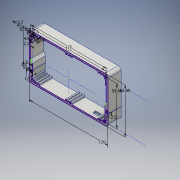
# Autodesk Inventor part: SZOMK-AK-C-C39
Saved by Autodesk Inventor 2016 (Build 200138000, 138)
## iProperties
Created: 2016-04-01
Part Number: SZOMK-AK-C-C39
Material: Aluminum 6061
Document SubType Name: Modeling
Designer: admin
Density: 2.7 g/cm^3
Appearance: Aluminum - Flat
Author: admin
Autodesk Inventor part; units mm, degrees
ref_plane "YZ Plane" through (0, 0, 0) normal (1, 0, 0) x (0, 1, 0)
ref_plane "XZ Plane" through (0, 0, 0) normal (0, 1, 0) x (-1, 0, 0)
ref_plane "XY Plane" through (0, 0, 0) normal (0, 0, 1) x (1, 0, 0)
sketch "Sketch1" plane through (0, 0, 0) normal (0, 1, 0) x (-1, 0, 0)
  arc A0 (55.1118, 28.4761) -> (54.0511, 29.5368) centre (55.5, 29.925) ccw
  arc A1 (-54.0059, 29.7916) -> (-55.1118, 28.4761) centre (-55.5, 29.925) ccw
  arc A2 (54.0511, -29.5368) -> (55.1118, -28.4761) centre (55.5, -29.925) ccw
  arc A3 (-55.1118, -28.4761) -> (-54.0511, -29.5368) centre (-55.5, -29.925) ccw
  line L0 (55.5, 34.425) -> (-55.5, 34.425)
  line L1 (55.5, -34.425) -> (-55.5, -34.425)
  line L2 (33.1179, 0) -> (-42.957, 0) construction
  line L3 (0, -20.0068) -> (0, 12.0803) construction
  line L4 (-77.7331, -29.925) -> (-117.8042, -29.925) construction
  line L5 (-91.6184, 29.925) -> (-122.9166, 29.925) construction
  line L6 (55.5, -18.8016) -> (55.5, 12.0803) construction
  line L7 (-55.5, -18.8016) -> (-55.5, 16.5996) construction
  arc A4 (55.5, -34.425) -> (60, -29.925) centre (55.5, -29.925) ccw
  arc A5 (60, 29.925) -> (55.5, 34.425) centre (55.5, 29.925) ccw
  arc A6 (-55.5, 34.425) -> (-60, 29.925) centre (-55.5, 29.925) ccw
  arc A7 (-60, -29.925) -> (-55.5, -34.425) centre (-55.5, -29.925) ccw
  line L8 (57.5, 27.125) -> (57.5, 25.125)
  line L9 (57.5, 25.125) -> (55.5, 25.125)
  line L10 (55.5, 25.125) -> (55.5, 23.125)
  line L11 (55.5, 23.125) -> (57.5, 23.125)
  line L12 (57.5, 23.125) -> (57.5, 21.125)
  line L13 (57.5, 21.125) -> (55.5, 21.125)
  line L14 (55.5, 21.125) -> (55.5, 19.125)
  line L15 (55.5, 19.125) -> (57.8, 19.125)
  line L16 (57.8, 19.125) -> (57.8, -3.3607)
  line L17 (-57.5, 27.125) -> (-57.5, 25.125)
  line L18 (-57.5, 25.125) -> (-55.5, 25.125)
  line L19 (-55.5, 25.125) -> (-55.5, 23.125)
  line L20 (-55.5, 23.125) -> (-57.5, 23.125)
  line L21 (-57.5, 23.125) -> (-57.5, 21.125)
  line L22 (-57.5, 21.125) -> (-55.5, 21.125)
  line L23 (-55.5, 21.125) -> (-55.5, 19.125)
  line L24 (-55.5, 19.125) -> (-57.8, 19.125)
  line L25 (-57.8, 19.125) -> (-57.8, -3.3607)
  line L26 (57.5, 27.125) -> (54.9678, 27.125)
  line L27 (52.7, 29.3928) -> (52.7, 31.925)
  line L28 (52.7, 31.925) -> (50.7, 31.925)
  line L29 (50.7, 31.925) -> (50.7, 29.925)
  line L30 (50.7, 29.925) -> (48.7, 29.925)
  line L31 (48.7, 29.925) -> (48.7, 31.925)
  line L32 (48.7, 31.925) -> (46.7, 31.925)
  line L33 (46.7, 31.925) -> (46.7, 29.925)
  line L34 (46.7, 29.925) -> (44.7, 29.925)
  line L35 (44.7, 29.925) -> (44.7, 32.225)
  line L36 (44.7, 32.225) -> (5, 32.225)
  line L37 (5, 32.225) -> (5, 29.925)
  line L38 (5, 29.925) -> (3, 29.925)
  line L39 (3, 29.925) -> (3, 31.925)
  line L40 (3, 31.925) -> (1, 31.925)
  line L41 (1, 31.925) -> (1, 29.925)
  line L42 (1, 29.925) -> (-1, 29.925)
  line L43 (-1, 29.925) -> (-1, 31.925)
  line L44 (-1, 31.925) -> (-3, 31.925)
  line L45 (-3, 31.925) -> (-3, 29.925)
  line L46 (-3, 29.925) -> (-5, 29.925)
  line L47 (-5, 29.925) -> (-5, 32.225)
  line L48 (-5, 32.225) -> (-44.7, 32.225)
  line L49 (-44.7, 32.225) -> (-44.7, 29.925)
  line L50 (-44.7, 29.925) -> (-46.7, 29.925)
  line L51 (-46.7, 29.925) -> (-46.7, 32.225)
  line L52 (-46.7, 32.225) -> (-48.7, 32.225)
  line L53 (-48.7, 32.225) -> (-48.7, 29.925)
  line L54 (-48.7, 29.925) -> (-50.7, 29.925)
  line L55 (-50.7, 29.925) -> (-50.7, 32.225)
  line L56 (-50.7, 32.225) -> (-52.7, 32.225)
  line L57 (-52.7, 32.225) -> (-52.7, 29.6928)
  line L58 (-54.9678, 27.125) -> (-57.5, 27.125)
  line L59 (55.1118, 28.4761) -> (54.6142, 27.9786)
  line L60 (54.0511, 29.5368) -> (53.5536, 29.0392)
  line L61 (55.5, 29.925) -> (49.0175, 23.4425) construction
  arc A8 (52.7, 29.3928) -> (53.5536, 29.0392) centre (53.2, 29.3928) ccw
  arc A9 (54.6142, 27.9786) -> (54.9678, 27.125) centre (54.9678, 27.625) ccw
  line L62 (-55.1118, 28.4761) -> (-54.6142, 27.9786)
  line L63 (-54.0059, 29.7916) -> (-53.5536, 29.3392)
  arc A10 (-53.5536, 29.3392) -> (-52.7, 29.6928) centre (-53.2, 29.6928) ccw
  arc A11 (-54.9678, 27.125) -> (-54.6142, 27.9786) centre (-54.9678, 27.625) ccw
  line L64 (57.8, -3.3607) -> (55, -7.6074)
  line L65 (55, -7.6074) -> (55, -16.775)
  arc A12 (56.5, -18.525) -> (58.5, -18.525) centre (57.5, -19.275) ccw
  line L66 (58.5, -18.525) -> (58.5, -16.775)
  line L67 (56.5, -18.525) -> (56.5, -16.775)
  line L68 (55, -16.775) -> (56.5, -16.775)
  line L69 (58.5, -16.775) -> (60, -16.775)
  line L70 (57.5, -16.4962) -> (57.5, -11.7384) construction
  line L71 (-57.8, -3.3607) -> (-55, -7.6074)
  line L72 (-55, -7.6074) -> (-55, -16.775)
  arc A13 (-56.5, -15.025) -> (-58.5, -15.025) centre (-57.5, -14.275) ccw
  line L73 (-58.5, -15.025) -> (-58.5, -16.775)
  line L74 (-56.5, -15.025) -> (-56.5, -16.775)
  line L75 (-55, -16.775) -> (-56.5, -16.775)
  line L76 (-58.5, -16.775) -> (-60, -16.775)
  line L77 (-57.5, -20.9142) -> (-57.5, -16.6435) construction
  line L78 (44.7, -32.225) -> (5, -32.225)
  line L79 (5, -32.225) -> (5, -29.925)
  line L80 (5, -29.925) -> (3, -29.925)
  line L81 (3, -29.925) -> (3, -31.925)
  line L82 (3, -31.925) -> (1, -31.925)
  line L83 (1, -31.925) -> (1, -29.925)
  line L84 (1, -29.925) -> (-1, -29.925)
  line L85 (-1, -29.925) -> (-1, -31.925)
  line L86 (-1, -31.925) -> (-3, -31.925)
  line L87 (-3, -31.925) -> (-3, -29.925)
  line L88 (-3, -29.925) -> (-5, -29.925)
  line L89 (-5, -29.925) -> (-5, -32.225)
  line L90 (-5, -32.225) -> (-44.7, -32.225)
  line L91 (55, -17.425) -> (55, -25.125)
  line L92 (55, -25.125) -> (57.5, -25.125)
  line L93 (57.5, -25.125) -> (57.5, -27.125)
  line L94 (57.5, -27.125) -> (54.9678, -27.125)
  line L95 (52.7, -29.3928) -> (52.7, -31.925)
  line L96 (52.7, -31.925) -> (50.7, -31.925)
  line L97 (50.7, -31.925) -> (50.7, -29.925)
  line L98 (50.7, -29.925) -> (48.7, -29.925)
  line L99 (48.7, -29.925) -> (48.7, -31.925)
  line L100 (48.7, -31.925) -> (46.7, -31.925)
  line L101 (46.7, -31.925) -> (46.7, -29.925)
  line L102 (46.7, -29.925) -> (44.7, -29.925)
  line L103 (44.7, -29.925) -> (44.7, -32.225)
  line L104 (-44.7, -32.225) -> (-44.7, -29.925)
  line L105 (-44.7, -29.925) -> (-46.7, -29.925)
  line L106 (-46.7, -29.925) -> (-46.7, -31.925)
  line L107 (-46.7, -31.925) -> (-48.7, -31.925)
  line L108 (-48.7, -31.925) -> (-48.7, -29.925)
  line L109 (-48.7, -29.925) -> (-50.7, -29.925)
  line L110 (-50.7, -29.925) -> (-50.7, -31.925)
  line L111 (-50.7, -31.925) -> (-52.7, -31.925)
  line L112 (-52.7, -31.925) -> (-52.7, -29.3928)
  line L113 (-54.9678, -27.125) -> (-57.5, -27.125)
  line L114 (-57.5, -27.125) -> (-57.5, -25.125)
  line L115 (-57.5, -25.125) -> (-55, -25.125)
  line L116 (-55, -25.125) -> (-55, -17.425)
  line L117 (54.6142, -27.9786) -> (55.1118, -28.4761)
  line L118 (53.5536, -29.0392) -> (54.0511, -29.5368)
  arc A14 (54.9678, -27.125) -> (54.6142, -27.9786) centre (54.9678, -27.625) ccw
  arc A15 (53.5536, -29.0392) -> (52.7, -29.3928) centre (53.2, -29.3928) ccw
  line L119 (-54.0511, -29.5368) -> (-53.5536, -29.0392)
  line L120 (-55.1118, -28.4761) -> (-54.6142, -27.9786)
  arc A16 (-52.7, -29.3928) -> (-53.5536, -29.0392) centre (-53.2, -29.3928) ccw
  arc A17 (-54.6142, -27.9786) -> (-54.9678, -27.125) centre (-54.9678, -27.625) ccw
  line L121 (55, -17.425) -> (56.5, -17.425)
  line L122 (58.5, -17.425) -> (60, -17.425)
  line L123 (60, -29.925) -> (60, -17.425)
  line L124 (60, -16.775) -> (60, 29.925)
  line L125 (-55, -17.425) -> (-56.5, -17.425)
  line L126 (-56.5, -17.425) -> (-56.5, -16.775)
  line L127 (-58.5, -16.775) -> (-58.5, -17.425)
  line L128 (-58.5, -17.425) -> (-60, -17.425)
  line L129 (-60, -29.925) -> (-60, -17.425)
  line L130 (-60, -16.775) -> (-60, 29.925)
  point P0 (0, 0)
  dimension "d1" = 111
  dimension "d2" = 59.85
  dimension "d3" = 68.85
  dimension "d5" = 115
  dimension "d8" = 1.5
  dimension "d11" = 2
  dimension "d12" = 45
  dimension "d13" = 7.3
  dimension "d14" = 1
  dimension "d16" = 2.5
  dimension "d17" = 1.5
  dimension "d18" = 2.2
  dimension "d19" = 2.5
  dimension "d20" = 51.2
  dimension "d21" = 2
  dimension "d23" = 2.5
  dimension "d25" = 2.5
  dimension "d26" = 17
  dimension "d27" = 2.2
  dimension "d29" = 4.5
  dimension "d30" = 120
  dimension "d31" = 5
  constraints: 263 end point, 70 perpendicular, 43 point on line, 39 collinear, 36 point on circle, 32 equal length, 20 tangent, 18 centre point, 15 vertical, 13 horizontal, 11 equal radius, 9 parallel, 4 coincident, 2 horizontal alignment, 2 vertical alignment, 21 other
  measures "d1" distance of A1.centre A0.centre
  measures "d2" distance of A1.centre A3.centre
  measures "d3" distance between parallel lines of L0 L1
  measures "d5" distance between parallel lines of L17 L8
  measures "d8" distance between parallel lines of L60 L59
  measures "d11" distance of L11.end L12.end
  measures "d12" angle of L0 L61
  measures "d13" distance between parallel lines of L0 L26
  measures "d14" diameter of A8
  measures "d16" distance between parallel lines of L0 L28
  measures "d17" radius of A0
  measures "d18" distance between parallel lines of L0 L36
  measures "d19" diameter of A12
  measures "d20" distance between parallel lines of L0 L69
  measures "d21" distance between parallel lines of L66 L67
  measures "d23" distance from line of L69 A12.centre
  measures "d25" distance from line of A13.centre L76
  measures "d26" distance between parallel lines of L1 L122
  measures "d27" distance between parallel lines of L124 L16
  measures "d29" distance between parallel lines of L124 L14
  measures "d30" distance between parallel lines of L129 L123
  measures "d31" distance between parallel lines of L124 L65
extrude "Extrusion1" add sketch "Sketch1" along normal blind 20 contours A0 L60 A8 L27 L28 L29 L30 L31 L32 L33 L34 L35 L36 L37 L38 L39 L40 L41 L42 L43 L44 L45 L46 L47 L48 L49 L50 L51 L52 L53 L54 L55 L56 L57 A10 L63 A1 L62 A11 L58 L17 L18 L19 L20 L21 L22 L23 L24 L25 L71 L72 L75 L74 A13 L73 L76 L130 A6 L0 A5 L124 L69 L66 A12 L67 L68 L65 L64 L16 L15 L14 L13 L12 L11 L10 L9 L8 L26 A9 L59
extrude "Extrusion2" add sketch "Sketch1" along normal blind 20 separate body contours L67 A12 L66 L122 L123 A4 L1 A7 L129 L128 L127 L73 A13 L74 L126 L125 L116 L115 L114 L113 A17 L120 A3 L119 A16 L112 L111 L110 L109 L108 L107 L106 L105 L104 L90 L89 L88 L87 L86 L85 L84 L83 L82 L81 L80 L79 L78 L103 L102 L101 L100 L99 L98 L97 L96 L95 A15 L118 A2 L117 A14 L94 L93 L92 L91 L121
sketch "Sketch2" plane through (55.5, 0, -34.425) normal (0, 0, -1) x (-1, 0, 0)
  line L0 (0, 20) -> (111, 20) projected
  line L1 (-4.5, 0) -> (-4.5, 20) projected
  line L2 (16, 9.4) -> (16, 7.73) construction
  line L3 (16, 7.73) -> (16.56, 7.17) construction
  line L4 (16.56, 7.17) -> (16.56, 5.5) construction
  line L5 (16.56, 5.5) -> (23.14, 5.5) construction
  line L6 (23.14, 5.5) -> (23.14, 7.17) construction
  line L7 (23.14, 7.17) -> (23.7, 7.73) construction
  line L8 (23.7, 7.73) -> (23.7, 9.4) construction
  line L9 (23.7, 9.4) -> (16, 9.4) construction
  line L10 (19.85, 8.0168) -> (19.85, 5.3617) construction
  line L11 (15.5, 9.9) -> (15.5, 7.5229)
  line L12 (15.5, 7.5229) -> (16.06, 6.9629)
  line L13 (16.06, 6.9629) -> (16.06, 5)
  line L14 (16.06, 5) -> (23.64, 5)
  line L15 (23.64, 5) -> (23.64, 6.9629)
  line L16 (23.64, 6.9629) -> (24.2, 7.5229)
  line L17 (24.2, 7.5229) -> (24.2, 9.9)
  line L18 (24.2, 9.9) -> (15.5, 9.9)
  line L19 (19.4089, 7.45) -> (22.3995, 7.45) construction
  line L20 (0, 0) -> (111, 0) construction
  point P0 (55.5, 0)
  point P1 (19.85, 9.4)
  point P2 (19.85, 5.5)
  dimension "d36" = 7.7
  dimension "d37" = 3.9
  dimension "d38" = 0.5
  dimension "d39" = 0.5
  dimension "d41" = 20
  dimension "d42" = 5
  dimension "d43" = 6.58
  dimension "d44" = 0.5
  dimension "d46" = 0.5
  constraints: 36 end point, 8 perpendicular, 5 parallel, 4 vertical, 2 midpoint, 2 point on line, 1 horizontal, 6 other
  measures "d36" distance between parallel lines of L8 L2
  measures "d37" distance between parallel lines of L5 L9
  measures "d38" distance between parallel lines of L18 L9
  measures "d39" distance between parallel lines of L2 L11
  measures "d41" distance between parallel lines of L11 L1
  measures "d42" distance between parallel lines of L20 L14
  measures "d43" distance between parallel lines of L6 L4
  measures "d44" distance between parallel lines of L4 L13
  measures "d46" distance between parallel lines of L12 L3
extrude "Extrusion3" cut sketch "Sketch2" against normal up to next bodies 2
equation "\"d16\" = d15"
equation "\"d18\" = d6"
equation "\"d15\" = 2.5"
equation "\"d6\" = 2.2"
body "Solid1"
body "Solid2"
